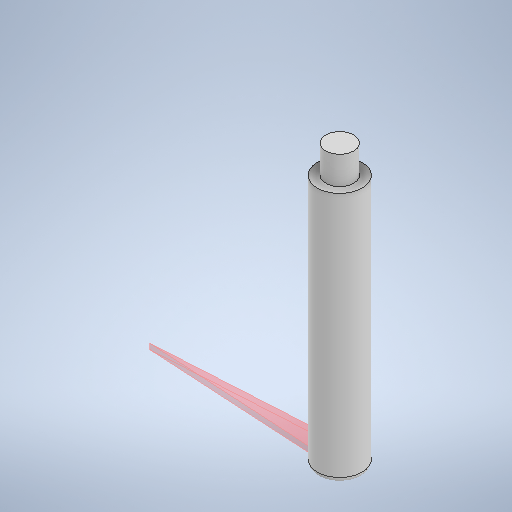
# Autodesk Inventor part: 202 part 3
Saved by Autodesk Inventor 2025.1 (Build 291241000, 241)
## iProperties
Created: 2024-09-02
Part Number: 202 part 3
Material: Generic
Document SubType Name: Modeling
Designer: ffogue
Density: 1 g/cm^3
Appearance: Default
Author: ffogue
Autodesk Inventor part; units mm, degrees
ref_plane "YZ Plane" through (0, 0, 0) normal (1, 0, 0) x (0, 1, 0)
ref_plane "XZ Plane" through (0, 0, 0) normal (0, 1, 0) x (-1, 0, 0)
sketch "Sketch1" plane through (0, 0, 0) normal (0, 0, 1) x (1, 0, 0)
  circle A0 centre (0, 0) radius 4
  circle A1 centre (0, 0) radius 2.5
  dimension "d0" = 8
  dimension "d19" = 5
  constraints: 2 centre point, 2 coincident
  measures "d0" diameter of A0
  measures "d19" diameter of A1
extrude "Extrusion4" add sketch "Sketch1" against normal blind 40 contours A0 | A1
extrude "Extrusion5" add sketch "Sketch1" against normal blind 45 contours A0 | A1
extrude "Extrusion6" add sketch "Sketch1" along normal blind 5 contours A1
ref_plane "Work Plane1" through (0, 0, -43) normal (0, 0, 1) x (1, 0, 0)
sketch "Sketch2" plane through (0, 0, -43) normal (0, 0, 1) x (1, 0, 0)
  circle A0 centre (0, 0) radius 4
  line L0 (-2.5, 2.5) -> (-2.5, -2.5)
  line L1 (-2.5, -2.5) -> (2.5, -2.5)
  line L2 (2.5, -2.5) -> (2.5, 2.5)
  line L3 (2.5, 2.5) -> (-2.5, 2.5)
  circle A1 centre (0, 0) radius 4
  line L4 (-3.6005, -1.7425) -> (-33.9574, 0)
  line L5 (-33.9574, 0) -> (-3.5932, 1.7575)
  line L6 (0, 0) -> (-33.6177, 0.0197) construction
  arc A2 (-3.5922, 1.7597) -> (-3.6005, -1.7425) centre (0.4698, -0.0011) ccw
  circle A3 centre (0, 0) radius 4
  circle A4 centre (0, 0) radius 4
  point P0 (-3.9574, 0.0094)
  point P1 (-3.5932, 1.7575)
  dimension "d9" = 30
  dimension "d10" = 3.5
  constraints: 6 centre point, 6 end point, 6 point on circle, 1 point on line
  measures "d9" distance of point (-3.957, 0.009) L4.end
  measures "d10" distance of L4.start L5.end
extrude "Extrusion3" add sketch "Sketch2" against normal blind 1 separate body contours L4 L5 A0
fillet "Fillet2" radius 1 1 edges at (-4, 0, -45)
body "Solid1"
body "Solid3"
